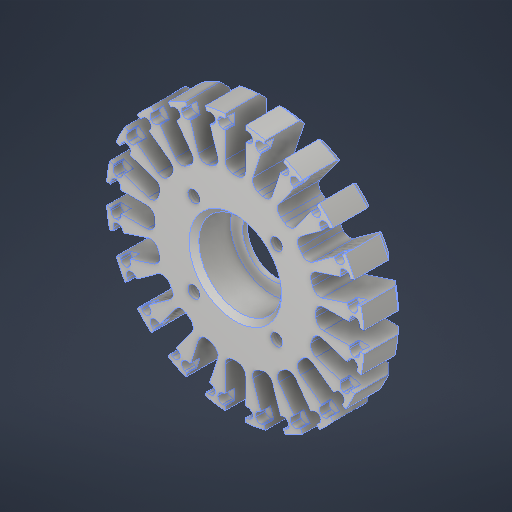
# Autodesk Inventor part: Radkasten
Saved by Autodesk Inventor 2025.2 (Build 292293000, 293)
## iProperties
Part Number: Radkasten
Material: Aluminium 6061
Document SubType Name: Modeling
Designer: rYan
Density: 2.7 g/cm^3
Appearance: Aluminium - flach
Mass: 11.5434 g
Surface Area: 96.0365 cm^2
Volume: 11.5434 cm^3
Author: rYan
Autodesk Inventor part; units mm, degrees
ref_plane "YZ Plane" through (0, 0, 0) normal (1, 0, 0) x (0, 1, 0)
ref_plane "XZ Plane" through (0, 0, 0) normal (0, 1, 0) x (-1, 0, 0)
ref_plane "XY Plane" through (0, 0, 0) normal (0, 0, 1) x (1, 0, 0)
sketch "Skizze1" plane through (0, 0, 0) normal (0, 0, 1) x (1, 0, 0)
  line L0 (0, 0) -> (0, 8.5)
  line L1 (4.75, 0) -> (4.75, 8.5)
  line L2 (4.75, 8.5) -> (5.8, 8.5)
  line L3 (5.8, 8.5) -> (5.8, 8.5)
  line L4 (21, 8.5) -> (26.5, 8.5)
  line L5 (26.5, 8.5) -> (26.5, 0)
  line L6 (26.5, 0) -> (4.75, 0)
  line L7 (-5.3, 0) -> (31.8, 0) projected
  line L8 (15.9, 8.5) -> (15.9, 8.5)
  line L9 (15.9, 8.5) -> (5.8, 8.5)
  line L10 (21, 8.5) -> (21, 8.5)
  line L11 (15.9, 8.5) -> (15.9, 8.5)
  line L12 (15.9, 8.5) -> (17.1, 8.5)
  line L13 (17.1, 8.5) -> (17.1, 8.5)
  line L14 (15.9, 8.5) -> (15.9, 8.5)
  line L15 (17.1, 8.5) -> (21, 8.5)
  line L16 (16.5, 8.5) -> (16.5, 0) construction
  dimension "d0" = 9.5
  dimension "d1" = 53
  dimension "d2" = 8.5
  dimension "d4" = 11.6
  dimension "d24" = 0
  dimension "d34" = 8.5
  dimension "d35" = 42
  dimension "d71" = 33
  dimension "d72" = 1.2
  dimension "d80" = 8.5
  constraints: 32 end point, 9 perpendicular, 4 point on line, 4 vertical, 3 horizontal, 2 midpoint, 1 collinear, 1 parallel
  measures "d0" diameter of L1 L0
  measures "d1" diameter of L5 L0
  measures "d2" distance of L4.end L5.end
  measures "d4" diameter of L3 L0
  measures "d24" distance of L8.start L8.end
  measures "d34" distance of L1.start L1.end
  measures "d35" diameter of L10 L0
  measures "d71" diameter of L16 L0
  measures "d72" distance of L11.end L12.end
  measures "d80" distance between parallel lines of L6 L12
revolve "Umdrehung1" add sketch "Skizze1" angle 360 about axis through (0, 0, 0) along (0, 1, 0)
sketch "Skizze2" plane through (0, 0, 0) normal (0, 1, 0) x (-1, 0, 0)
  circle A0 centre (0, 0) radius 26.5 projected
  circle A1 centre (0, 0) radius 16.5 construction
  line L0 (2.1, 26.5) -> (-2.1, 26.5)
  line L1 (-2.1, 26.5) -> (-2.1, 18.1)
  line L2 (-0.5, 16.5) -> (0.5, 16.5)
  line L3 (2.1, 18.1) -> (2.1, 26.5)
  line L4 (0, 0) -> (0, 26.5) construction
  arc A2 (0.5, 16.5) -> (2.1, 18.1) centre (0.5, 18.1) ccw
  arc A3 (-2.1, 18.1) -> (-0.5, 16.5) centre (-0.5, 18.1) ccw
  dimension "d6" = 1.6
  dimension "d7" = 4.2
  dimension "d8" = 33
  constraints: 10 end point, 5 tangent, 4 point on circle, 3 centre point, 2 parallel, 1 coincident, 1 equal radius, 1 horizontal, 1 midpoint, 1 perpendicular, 1 vertical, 1 vertical alignment, 2 other
  measures "d6" radius of A2
  measures "d7" distance between parallel lines of L1 L3
  measures "d8" diameter of A1
extrude "Querrolle" cut sketch "Skizze2" along normal blind 8.5 contours L3 A2 L2 A3 L1 A0 | A0 L0 L3 | L1 L0 A0 picked at (0, 20.9)
sketch "Skizze3" plane through (0, 0, 0) normal (0, 1, 0) x (-1, 0, 0)
  line L0 (2.6, 25.525) -> (-2.6, 25.525)
  line L1 (-3.6, 24.525) -> (-3.6, 24.475)
  line L2 (-2.6, 23.475) -> (2.6, 23.475)
  line L3 (3.6, 24.475) -> (3.6, 24.525)
  line L4 (0, -5.2833) -> (0, 31.7) projected
  line L5 (2.65, 25.504) -> (-2.65, 25.504) construction
  line L6 (-2.65, 25.504) -> (-2.65, 23.496) construction
  line L7 (-2.65, 23.496) -> (2.65, 23.496) construction
  line L8 (2.65, 23.496) -> (2.65, 25.504) construction
  line L9 (-2.65, 25.504) -> (-3, 25.4102) construction
  line L10 (-3, 25.4102) -> (-3, 23.5898) construction
  line L11 (-3, 23.5898) -> (-2.65, 23.496) construction
  line L12 (2.65, 25.504) -> (3, 25.4102) construction
  line L13 (3, 25.4102) -> (3, 23.5898) construction
  line L14 (3, 23.5898) -> (2.65, 23.496) construction
  line L15 (3, 24.5) -> (-3, 24.5) construction
  line L16 (0, 25.504) -> (0, 23.496) construction
  arc A0 (3.6, 24.525) -> (2.6, 25.525) centre (2.6, 24.525) ccw
  arc A1 (-2.6, 25.525) -> (-3.6, 24.525) centre (-2.6, 24.525) ccw
  arc A2 (-3.6, 24.475) -> (-2.6, 23.475) centre (-2.6, 24.475) ccw
  arc A3 (2.6, 23.475) -> (3.6, 24.475) centre (2.6, 24.475) ccw
  line L17 (3.6, 24.5) -> (-3.6, 24.5) construction
  line L18 (2.1, 18.1) -> (2.1, 26.4167) projected
  line L19 (3.375, 24.75) -> (2.6, 25.525) construction
  line L20 (2.6, 25.525) -> (-2.6, 25.525) construction
  line L21 (-2.6, 25.525) -> (-3.375, 24.75) construction
  line L22 (-3.375, 24.75) -> (-3.375, 24.5) construction
  line L23 (3.375, 24.75) -> (3.375, 24.5) construction
  line L24 (0, 24.5) -> (0, 31.35)
  circle A4 centre (0, 0) radius 31.35
  point P0 (3.6, 25.525)
  point P1 (-3.6, 25.525)
  point P2 (2.65, 24.5)
  point P3 (-2.65, 24.5)
  point P4 (0, 24.5)
  point P5 (2.1, 26.2538)
  dimension "d11" = 2.05
  dimension "d12" = 7.2
  dimension "d13" = 2.008
  dimension "d14" = 15
  dimension "d15" = 0.35
  dimension "d16" = 6
  dimension "d17" = 1
  dimension "d18" = 24.5
  dimension "d82" = 0.55
  dimension "d83" = 0.5
  dimension "d84" = 45
  dimension "d85" = 1.025
  dimension "d86" = 0.5
  dimension "d87" = 0.25
  dimension "d236" = 6.85
  constraints: 46 end point, 11 midpoint, 10 point on line, 8 point on circle, 8 tangent, 5 parallel, 4 centre point, 4 perpendicular, 3 equal radius, 3 horizontal, 1 coincident, 1 vertical, 1 vertical alignment, 8 other
  measures "d11" distance between parallel lines of L0 L2
  measures "d12" distance of point (3.6, 25.525) point (-3.6, 25.525)
  measures "d13" distance between parallel lines of L7 L5
  measures "d14" angle of L5 L9
  measures "d15" distance between parallel lines of L6 L10
  measures "d16" distance between parallel lines of L10 L13
  measures "d17" radius of A0
  measures "d18" distance from line of L17 point (0, 0)
  measures "d82" distance from line of L5.start L18
  measures "d83" distance from line of L0.start L18
  measures "d84" angle of L20 L21
  measures "d85" distance between parallel lines of L15 L20
  measures "d86" distance from line of L18 L19.end
  measures "d87" distance from line of L17 L19.start
  measures "d236" distance of L24.start L24.end
extrude "Achse" cut sketch "Skizze3" along normal blind 2 contours A0 L3 A3 L2 L18 L0 | L18 L2 L4 L0 | L4 L2 A2 L1 A1 L0
fillet "Rundung1" radius 0.1 4 edges at (-2.1, 1, 25.525) (-2.1, 1, 23.475) (2.1, 1, 25.525) (2.1, 1, 23.475)
pattern_circular "Runde Anordnung1" count 20 over 360 about axis through (0, -10, 0) along (0, 1, 0) of "Querrolle", "Achse", "Rundung1"
sketch "Skizze6" plane through (0.25, 8.5, 18) normal (0, -1, 0) x (0.7071068, 0, -0.7071068)
  circle A0 centre (12.5511, -12.9047) radius 8.5 construction
  line L0 (4.0511, -12.9047) -> (21.0511, -12.9047) construction
  line L1 (12.5511, -21.4047) -> (12.5511, -4.4047) construction
  dimension "d48" = 17
  constraints: 5 coincident, 4 end point, 4 midpoint, 4 point on circle, 1 centre point, 1 horizontal, 1 perpendicular
  measures "d48" diameter of A0
hole "Fräshilfe" [suppressed]
chamfer "Fasen" distance 1.5 angle 45 20 edges at (23.6117, 8.5, -12.0307) (18.7383, 8.5, -18.7383) (12.0307, 8.5, -23.6117) (4.1455, 8.5, -26.1737) (-4.1455, 8.5, -26.1737) (-12.0307, 8.5, -23.6117) (-18.7383, 8.5, -18.7383) (-23.6117, 8.5, -12.0307) (-26.1737, 8.5, -4.1455) (-26.1737, 8.5, 4.1455) (-23.6117, 8.5, 12.0307) (-18.7383, 8.5, 18.7383) (-12.0307, 8.5, 23.6117) (-4.1455, 8.5, 26.1737) (4.1455, 8.5, 26.1737) (12.0307, 8.5, 23.6117) (18.7383, 8.5, 18.7383) (23.6117, 8.5, 12.0307) (26.1737, 8.5, 4.1455) (26.1737, 8.5, -4.1455)
sketch "Skizze22" plane through (-24.9116, 8.5, -2.1) normal (0, 1, 0) x (1, 0, 0)
  line L0 (25.4822, 13.5146) -> (25.1616, 12.3978)
  arc A0 (25.1616, 12.3978) -> (24.6616, 12.3978) centre (24.9116, -2.1) ccw
  line L1 (24.6616, 12.3978) -> (24.3411, 13.5146)
  arc A1 (24.3411, 13.5146) -> (23.8469, 13.4887) centre (24.9116, -2.1) ccw
  line L2 (23.8469, 13.4887) -> (23.6448, 12.3446)
  arc A2 (23.6448, 12.3446) -> (23.1476, 12.2923) centre (24.9116, -2.1) ccw
  line L3 (23.1476, 12.2923) -> (22.7121, 13.3694)
  arc A3 (22.7121, 13.3694) -> (22.2233, 13.292) centre (24.9116, -2.1) ccw
  line L4 (22.2233, 13.292) -> (22.1419, 12.133)
  arc A4 (22.1419, 12.133) -> (21.6528, 12.0291) centre (24.9116, -2.1) ccw
  line L5 (21.6528, 12.0291) -> (21.1071, 13.0547)
  arc A5 (21.1071, 13.0547) -> (20.6291, 12.9267) centre (24.9116, -2.1) ccw
  line L6 (20.6291, 12.9267) -> (20.6693, 11.7655)
  arc A6 (20.6693, 11.7655) -> (20.1938, 11.611) centre (24.9116, -2.1) ccw
  line L7 (20.1938, 11.611) -> (19.5439, 12.574)
  arc A7 (19.5439, 12.574) -> (19.0818, 12.3967) centre (24.9116, -2.1) ccw
  line L8 (19.0818, 12.3967) -> (19.2432, 11.2461)
  arc A8 (19.2432, 11.2461) -> (18.7865, 11.0428) centre (24.9116, -2.1) ccw
  line L9 (18.7865, 11.0428) -> (18.0394, 11.9326)
  arc A9 (18.0394, 11.9326) -> (17.5984, 11.7079) centre (24.9116, -2.1) ccw
  line L10 (17.5984, 11.7079) -> (17.8792, 10.5805)
  arc A10 (17.8792, 10.5805) -> (17.4462, 10.3305) centre (24.9116, -2.1) ccw
  line L11 (17.4462, 10.3305) -> (16.6103, 11.1374)
  arc A11 (16.6103, 11.1374) -> (16.1952, 10.8678) centre (24.9116, -2.1) ccw
  line L12 (16.1952, 10.8678) -> (16.5923, 9.7759)
  arc A12 (16.5923, 9.7759) -> (16.1878, 9.4821) centre (24.9116, -2.1) ccw
  line L13 (16.1878, 9.4821) -> (15.2721, 10.1971)
  arc A13 (15.2721, 10.1971) -> (14.8874, 9.8857) centre (24.9116, -2.1) ccw
  line L14 (14.8874, 9.8857) -> (15.3965, 8.8413)
  arc A14 (15.3965, 8.8413) -> (15.0249, 8.5067) centre (24.9116, -2.1) ccw
  line L15 (15.0249, 8.5067) -> (14.0395, 9.1221)
  arc A15 (14.0395, 9.1221) -> (13.6895, 8.7722) centre (24.9116, -2.1) ccw
  line L16 (13.6895, 8.7722) -> (14.3049, 7.7867)
  arc A16 (14.3049, 7.7867) -> (13.9704, 7.4152) centre (24.9116, -2.1) ccw
  line L17 (13.9704, 7.4152) -> (12.926, 7.9242)
  arc A17 (12.926, 7.9242) -> (12.6145, 7.5396) centre (24.9116, -2.1) ccw
  line L18 (12.6145, 7.5396) -> (13.3296, 6.6239)
  arc A18 (13.3296, 6.6239) -> (13.0357, 6.2194) centre (24.9116, -2.1) ccw
  line L19 (13.0357, 6.2194) -> (11.9438, 6.6165)
  arc A19 (11.9438, 6.6165) -> (11.6743, 6.2014) centre (24.9116, -2.1) ccw
  line L20 (11.6743, 6.2014) -> (12.4811, 5.3654)
  arc A20 (12.4811, 5.3654) -> (12.2311, 4.9324) centre (24.9116, -2.1) ccw
  line L21 (12.2311, 4.9324) -> (11.1038, 5.2132)
  arc A21 (11.1038, 5.2132) -> (10.8791, 4.7722) centre (24.9116, -2.1) ccw
  line L22 (10.8791, 4.7722) -> (11.7689, 4.0252)
  arc A22 (11.7689, 4.0252) -> (11.5655, 3.5684) centre (24.9116, -2.1) ccw
  line L23 (11.5655, 3.5684) -> (10.415, 3.7298)
  arc A23 (10.415, 3.7298) -> (10.2376, 3.2678) centre (24.9116, -2.1) ccw
  line L24 (10.2376, 3.2678) -> (11.2006, 2.6178)
  arc A24 (11.2006, 2.6178) -> (11.0461, 2.1423) centre (24.9116, -2.1) ccw
  line L25 (11.0461, 2.1423) -> (9.885, 2.1826)
  arc A25 (9.885, 2.1826) -> (9.7569, 1.7045) centre (24.9116, -2.1) ccw
  line L26 (9.7569, 1.7045) -> (10.7826, 1.1588)
  arc A26 (10.7826, 1.1588) -> (10.6786, 0.6697) centre (24.9116, -2.1) ccw
  line L27 (10.6786, 0.6697) -> (9.5197, 0.5884)
  arc A27 (9.5197, 0.5884) -> (9.4422, 0.0996) centre (24.9116, -2.1) ccw
  line L28 (9.4422, 0.0996) -> (10.5194, -0.3359)
  arc A28 (10.5194, -0.3359) -> (10.4671, -0.8332) centre (24.9116, -2.1) ccw
  line L29 (10.4671, -0.8332) -> (9.323, -1.0352)
  arc A29 (9.323, -1.0352) -> (9.2971, -1.5295) centre (24.9116, -2.1) ccw
  line L30 (9.2971, -1.5295) -> (10.4138, -1.85)
  arc A30 (10.4138, -1.85) -> (10.4138, -2.35) centre (24.9116, -2.1) ccw
  line L31 (10.4138, -2.35) -> (9.2971, -2.6705)
  arc A31 (9.2971, -2.6705) -> (9.323, -3.1648) centre (24.9116, -2.1) ccw
  line L32 (9.323, -3.1648) -> (10.4671, -3.3668)
  arc A32 (10.4671, -3.3668) -> (10.5194, -3.8641) centre (24.9116, -2.1) ccw
  line L33 (10.5194, -3.8641) -> (9.4422, -4.2996)
  arc A33 (9.4422, -4.2996) -> (9.5197, -4.7884) centre (24.9116, -2.1) ccw
  line L34 (9.5197, -4.7884) -> (10.6786, -4.8697)
  arc A34 (10.6786, -4.8697) -> (10.7826, -5.3588) centre (24.9116, -2.1) ccw
  line L35 (10.7826, -5.3588) -> (9.7569, -5.9045)
  arc A35 (9.7569, -5.9045) -> (9.885, -6.3826) centre (24.9116, -2.1) ccw
  line L36 (9.885, -6.3826) -> (11.0461, -6.3423)
  arc A36 (11.0461, -6.3423) -> (11.2006, -6.8178) centre (24.9116, -2.1) ccw
  line L37 (11.2006, -6.8178) -> (10.2376, -7.4678)
  arc A37 (10.2376, -7.4678) -> (10.415, -7.9298) centre (24.9116, -2.1) ccw
  line L38 (10.415, -7.9298) -> (11.5655, -7.7684)
  arc A38 (11.5655, -7.7684) -> (11.7689, -8.2252) centre (24.9116, -2.1) ccw
  line L39 (11.7689, -8.2252) -> (10.8791, -8.9722)
  arc A39 (10.8791, -8.9722) -> (11.1038, -9.4132) centre (24.9116, -2.1) ccw
  line L40 (11.1038, -9.4132) -> (12.2311, -9.1324)
  arc A40 (12.2311, -9.1324) -> (12.4811, -9.5654) centre (24.9116, -2.1) ccw
  line L41 (12.4811, -9.5654) -> (11.6743, -10.4014)
  arc A41 (11.6743, -10.4014) -> (11.9438, -10.8165) centre (24.9116, -2.1) ccw
  line L42 (11.9438, -10.8165) -> (13.0357, -10.4194)
  arc A42 (13.0357, -10.4194) -> (13.3296, -10.8239) centre (24.9116, -2.1) ccw
  line L43 (13.3296, -10.8239) -> (12.6145, -11.7396)
  arc A43 (12.6145, -11.7396) -> (12.926, -12.1242) centre (24.9116, -2.1) ccw
  line L44 (12.926, -12.1242) -> (13.9704, -11.6152)
  arc A44 (13.9704, -11.6152) -> (14.3049, -11.9867) centre (24.9116, -2.1) ccw
  line L45 (14.3049, -11.9867) -> (13.6895, -12.9722)
  arc A45 (13.6895, -12.9722) -> (14.0395, -13.3221) centre (24.9116, -2.1) ccw
  line L46 (14.0395, -13.3221) -> (15.0249, -12.7067)
  arc A46 (15.0249, -12.7067) -> (15.3965, -13.0413) centre (24.9116, -2.1) ccw
  line L47 (15.3965, -13.0413) -> (14.8874, -14.0857)
  arc A47 (14.8874, -14.0857) -> (15.2721, -14.3971) centre (24.9116, -2.1) ccw
  line L48 (15.2721, -14.3971) -> (16.1878, -13.6821)
  arc A48 (16.1878, -13.6821) -> (16.5923, -13.9759) centre (24.9116, -2.1) ccw
  line L49 (16.5923, -13.9759) -> (16.1952, -15.0678)
  arc A49 (16.1952, -15.0678) -> (16.6103, -15.3374) centre (24.9116, -2.1) ccw
  line L50 (16.6103, -15.3374) -> (17.4462, -14.5305)
  arc A50 (17.4462, -14.5305) -> (17.8792, -14.7805) centre (24.9116, -2.1) ccw
  line L51 (17.8792, -14.7805) -> (17.5984, -15.9079)
  arc A51 (17.5984, -15.9079) -> (18.0394, -16.1326) centre (24.9116, -2.1) ccw
  line L52 (18.0394, -16.1326) -> (18.7865, -15.2428)
  arc A52 (18.7865, -15.2428) -> (19.2432, -15.4461) centre (24.9116, -2.1) ccw
  line L53 (19.2432, -15.4461) -> (19.0818, -16.5967)
  arc A53 (19.0818, -16.5967) -> (19.5439, -16.774) centre (24.9116, -2.1) ccw
  line L54 (19.5439, -16.774) -> (20.1938, -15.811)
  arc A54 (20.1938, -15.811) -> (20.6693, -15.9655) centre (24.9116, -2.1) ccw
  line L55 (20.6693, -15.9655) -> (20.6291, -17.1267)
  arc A55 (20.6291, -17.1267) -> (21.1071, -17.2547) centre (24.9116, -2.1) ccw
  line L56 (21.1071, -17.2547) -> (21.6528, -16.2291)
  arc A56 (21.6528, -16.2291) -> (22.1419, -16.333) centre (24.9116, -2.1) ccw
  line L57 (22.1419, -16.333) -> (22.2233, -17.492)
  arc A57 (22.2233, -17.492) -> (22.7121, -17.5694) centre (24.9116, -2.1) ccw
  line L58 (22.7121, -17.5694) -> (23.1476, -16.4923)
  arc A58 (23.1476, -16.4923) -> (23.6448, -16.5446) centre (24.9116, -2.1) ccw
  line L59 (23.6448, -16.5446) -> (23.8469, -17.6887)
  arc A59 (23.8469, -17.6887) -> (24.3411, -17.7146) centre (24.9116, -2.1) ccw
  line L60 (24.3411, -17.7146) -> (24.6616, -16.5978)
  arc A60 (24.6616, -16.5978) -> (25.1616, -16.5978) centre (24.9116, -2.1) ccw
  line L61 (25.1616, -16.5978) -> (25.4822, -17.7146)
  arc A61 (25.4822, -17.7146) -> (25.9764, -17.6887) centre (24.9116, -2.1) ccw
  line L62 (25.9764, -17.6887) -> (26.1785, -16.5446)
  arc A62 (26.1785, -16.5446) -> (26.6757, -16.4923) centre (24.9116, -2.1) ccw
  line L63 (26.6757, -16.4923) -> (27.1112, -17.5694)
  arc A63 (27.1112, -17.5694) -> (27.6, -17.492) centre (24.9116, -2.1) ccw
  line L64 (27.6, -17.492) -> (27.6814, -16.333)
  arc A64 (27.6814, -16.333) -> (28.1705, -16.2291) centre (24.9116, -2.1) ccw
  line L65 (28.1705, -16.2291) -> (28.7162, -17.2547)
  arc A65 (28.7162, -17.2547) -> (29.1942, -17.1267) centre (24.9116, -2.1) ccw
  line L66 (29.1942, -17.1267) -> (29.154, -15.9655)
  arc A66 (29.154, -15.9655) -> (29.6295, -15.811) centre (24.9116, -2.1) ccw
  line L67 (29.6295, -15.811) -> (30.2794, -16.774)
  arc A67 (30.2794, -16.774) -> (30.7415, -16.5967) centre (24.9116, -2.1) ccw
  line L68 (30.7415, -16.5967) -> (30.5801, -15.4461)
  arc A68 (30.5801, -15.4461) -> (31.0368, -15.2428) centre (24.9116, -2.1) ccw
  line L69 (31.0368, -15.2428) -> (31.7839, -16.1326)
  arc A69 (31.7839, -16.1326) -> (32.2248, -15.9079) centre (24.9116, -2.1) ccw
  line L70 (32.2248, -15.9079) -> (31.9441, -14.7805)
  arc A70 (31.9441, -14.7805) -> (32.3771, -14.5305) centre (24.9116, -2.1) ccw
  line L71 (32.3771, -14.5305) -> (33.213, -15.3374)
  arc A71 (33.213, -15.3374) -> (33.6281, -15.0678) centre (24.9116, -2.1) ccw
  line L72 (33.6281, -15.0678) -> (33.231, -13.9759)
  arc A72 (33.231, -13.9759) -> (33.6355, -13.6821) centre (24.9116, -2.1) ccw
  line L73 (33.6355, -13.6821) -> (34.5512, -14.3971)
  arc A73 (34.5512, -14.3971) -> (34.9359, -14.0857) centre (24.9116, -2.1) ccw
  line L74 (34.9359, -14.0857) -> (34.4268, -13.0413)
  arc A74 (34.4268, -13.0413) -> (34.7984, -12.7067) centre (24.9116, -2.1) ccw
  line L75 (34.7984, -12.7067) -> (35.7838, -13.3221)
  arc A75 (35.7838, -13.3221) -> (36.1338, -12.9722) centre (24.9116, -2.1) ccw
  line L76 (36.1338, -12.9722) -> (35.5184, -11.9867)
  arc A76 (35.5184, -11.9867) -> (35.8529, -11.6152) centre (24.9116, -2.1) ccw
  line L77 (35.8529, -11.6152) -> (36.8973, -12.1242)
  arc A77 (36.8973, -12.1242) -> (37.2088, -11.7396) centre (24.9116, -2.1) ccw
  line L78 (37.2088, -11.7396) -> (36.4937, -10.8239)
  arc A78 (36.4937, -10.8239) -> (36.7876, -10.4194) centre (24.9116, -2.1) ccw
  line L79 (36.7876, -10.4194) -> (37.8795, -10.8165)
  arc A79 (37.8795, -10.8165) -> (38.149, -10.4014) centre (24.9116, -2.1) ccw
  line L80 (38.149, -10.4014) -> (37.3421, -9.5654)
  arc A80 (37.3421, -9.5654) -> (37.5921, -9.1324) centre (24.9116, -2.1) ccw
  line L81 (37.5921, -9.1324) -> (38.7195, -9.4132)
  arc A81 (38.7195, -9.4132) -> (38.9442, -8.9722) centre (24.9116, -2.1) ccw
  line L82 (38.9442, -8.9722) -> (38.0544, -8.2252)
  arc A82 (38.0544, -8.2252) -> (38.2578, -7.7684) centre (24.9116, -2.1) ccw
  line L83 (38.2578, -7.7684) -> (39.4083, -7.9298)
  arc A83 (39.4083, -7.9298) -> (39.5857, -7.4678) centre (24.9116, -2.1) ccw
  line L84 (39.5857, -7.4678) -> (38.6227, -6.8178)
  arc A84 (38.6227, -6.8178) -> (38.7772, -6.3423) centre (24.9116, -2.1) ccw
  line L85 (38.7772, -6.3423) -> (39.9383, -6.3826)
  arc A85 (39.9383, -6.3826) -> (40.0664, -5.9045) centre (24.9116, -2.1) ccw
  line L86 (40.0664, -5.9045) -> (39.0407, -5.3588)
  arc A86 (39.0407, -5.3588) -> (39.1447, -4.8697) centre (24.9116, -2.1) ccw
  line L87 (39.1447, -4.8697) -> (40.3036, -4.7884)
  arc A87 (40.3036, -4.7884) -> (40.381, -4.2996) centre (24.9116, -2.1) ccw
  line L88 (40.381, -4.2996) -> (39.3039, -3.8641)
  arc A88 (39.3039, -3.8641) -> (39.3562, -3.3668) centre (24.9116, -2.1) ccw
  line L89 (39.3562, -3.3668) -> (40.5003, -3.1648)
  arc A89 (40.5003, -3.1648) -> (40.5262, -2.6705) centre (24.9116, -2.1) ccw
  line L90 (40.5262, -2.6705) -> (39.4095, -2.35)
  arc A90 (39.4095, -2.35) -> (39.4095, -1.85) centre (24.9116, -2.1) ccw
  line L91 (39.4095, -1.85) -> (40.5262, -1.5295)
  arc A91 (40.5262, -1.5295) -> (40.5003, -1.0352) centre (24.9116, -2.1) ccw
  line L92 (40.5003, -1.0352) -> (39.3562, -0.8332)
  arc A92 (39.3562, -0.8332) -> (39.3039, -0.3359) centre (24.9116, -2.1) ccw
  line L93 (39.3039, -0.3359) -> (40.381, 0.0996)
  arc A93 (40.381, 0.0996) -> (40.3036, 0.5884) centre (24.9116, -2.1) ccw
  line L94 (40.3036, 0.5884) -> (39.1447, 0.6697)
  arc A94 (39.1447, 0.6697) -> (39.0407, 1.1588) centre (24.9116, -2.1) ccw
  line L95 (39.0407, 1.1588) -> (40.0664, 1.7045)
  arc A95 (40.0664, 1.7045) -> (39.9383, 2.1826) centre (24.9116, -2.1) ccw
  line L96 (39.9383, 2.1826) -> (38.7772, 2.1423)
  arc A96 (38.7772, 2.1423) -> (38.6227, 2.6178) centre (24.9116, -2.1) ccw
  line L97 (38.6227, 2.6178) -> (39.5857, 3.2678)
  arc A97 (39.5857, 3.2678) -> (39.4083, 3.7298) centre (24.9116, -2.1) ccw
  line L98 (39.4083, 3.7298) -> (38.2578, 3.5684)
  arc A98 (38.2578, 3.5684) -> (38.0544, 4.0252) centre (24.9116, -2.1) ccw
  line L99 (38.0544, 4.0252) -> (38.9442, 4.7722)
  arc A99 (38.9442, 4.7722) -> (38.7195, 5.2132) centre (24.9116, -2.1) ccw
  line L100 (38.7195, 5.2132) -> (37.5921, 4.9324)
  arc A100 (37.5921, 4.9324) -> (37.3421, 5.3654) centre (24.9116, -2.1) ccw
  line L101 (37.3421, 5.3654) -> (38.149, 6.2014)
  arc A101 (38.149, 6.2014) -> (37.8795, 6.6165) centre (24.9116, -2.1) ccw
  line L102 (37.8795, 6.6165) -> (36.7876, 6.2194)
  arc A102 (36.7876, 6.2194) -> (36.4937, 6.6239) centre (24.9116, -2.1) ccw
  line L103 (36.4937, 6.6239) -> (37.2088, 7.5396)
  arc A103 (37.2088, 7.5396) -> (36.8973, 7.9242) centre (24.9116, -2.1) ccw
  line L104 (36.8973, 7.9242) -> (35.8529, 7.4152)
  arc A104 (35.8529, 7.4152) -> (35.5184, 7.7867) centre (24.9116, -2.1) ccw
  line L105 (35.5184, 7.7867) -> (36.1338, 8.7722)
  arc A105 (36.1338, 8.7722) -> (35.7838, 9.1221) centre (24.9116, -2.1) ccw
  line L106 (35.7838, 9.1221) -> (34.7984, 8.5067)
  arc A106 (34.7984, 8.5067) -> (34.4268, 8.8413) centre (24.9116, -2.1) ccw
  line L107 (34.4268, 8.8413) -> (34.9359, 9.8857)
  arc A107 (34.9359, 9.8857) -> (34.5512, 10.1971) centre (24.9116, -2.1) ccw
  line L108 (34.5512, 10.1971) -> (33.6355, 9.4821)
  arc A108 (33.6355, 9.4821) -> (33.231, 9.7759) centre (24.9116, -2.1) ccw
  line L109 (33.231, 9.7759) -> (33.6281, 10.8678)
  arc A109 (33.6281, 10.8678) -> (33.213, 11.1374) centre (24.9116, -2.1) ccw
  line L110 (33.213, 11.1374) -> (32.3771, 10.3305)
  arc A110 (32.3771, 10.3305) -> (31.9441, 10.5805) centre (24.9116, -2.1) ccw
  line L111 (31.9441, 10.5805) -> (32.2248, 11.7079)
  arc A111 (32.2248, 11.7079) -> (31.7839, 11.9326) centre (24.9116, -2.1) ccw
  line L112 (31.7839, 11.9326) -> (31.0368, 11.0428)
  arc A112 (31.0368, 11.0428) -> (30.5801, 11.2461) centre (24.9116, -2.1) ccw
  line L113 (30.5801, 11.2461) -> (30.7415, 12.3967)
  arc A113 (30.7415, 12.3967) -> (30.2794, 12.574) centre (24.9116, -2.1) ccw
  line L114 (30.2794, 12.574) -> (29.6295, 11.611)
  arc A114 (29.6295, 11.611) -> (29.154, 11.7655) centre (24.9116, -2.1) ccw
  line L115 (29.154, 11.7655) -> (29.1942, 12.9267)
  arc A115 (29.1942, 12.9267) -> (28.7162, 13.0547) centre (24.9116, -2.1) ccw
  line L116 (28.7162, 13.0547) -> (28.1705, 12.0291)
  arc A116 (28.1705, 12.0291) -> (27.6814, 12.133) centre (24.9116, -2.1) ccw
  line L117 (27.6814, 12.133) -> (27.6, 13.292)
  arc A117 (27.6, 13.292) -> (27.1112, 13.3694) centre (24.9116, -2.1) ccw
  line L118 (27.1112, 13.3694) -> (26.6757, 12.2923)
  arc A118 (26.6757, 12.2923) -> (26.1785, 12.3446) centre (24.9116, -2.1) ccw
  line L119 (26.1785, 12.3446) -> (25.9764, 13.4887)
  arc A119 (25.9764, 13.4887) -> (25.4822, 13.5146) centre (24.9116, -2.1) ccw
  point P0 (24.9116, -2.1)
  point P1 (24.9116, -2.1)
  point P2 (48.0004, 1.5569)
  point P3 (21.2547, 20.9887)
  point P4 (1.8229, -5.7569)
  point P5 (28.5685, -25.1887)
  dimension "d207" = 360
  constraints: 240 end point, 240 point on circle, 120 centre point, 5 other
hole "Bohrung4" at (23.0887, 8.5, -3.6569) at (-3.6569, 8.5, -23.0887) at (-23.0887, 8.5, 3.6569) at (3.6569, 8.5, 23.0887) direction (0, -1, 0) diameter 1.567 depth 4 tip angle 118 thread size "M2x0.4" class "6H" standard "ISO Metric profile"
sketch "Skizze23" plane through (0.5, 0, 18.1) normal (0, -1, 0) x (0.7071068, 0, -0.7071068)
  circle A0 centre (12.4451, -13.1522) radius 7.05
  dimension "d216" = 14.1
  constraints: 1 centre point, 1 coincident
  measures "d216" diameter of A0
extrude "Extrusion16" cut sketch "Skizze23" against normal blind 7.5
sketch "Skizze24" plane through (0.5, 0, 18.1) normal (0, -1, 0) x (0.7071068, 0, -0.7071068)
  circle A0 centre (12.4451, -13.1522) radius 8.5
  dimension "d219" = 17
  constraints: 1 centre point, 1 coincident
  measures "d219" diameter of A0
extrude "Extrusion17" cut sketch "Skizze24" against normal blind 7.5
chamfer "Fasen26" distance 1 angle 45 1 edges at (-6.0104, 0, 6.0104)
sketch "Skizze25" plane through (0.5, 0, 18.1) normal (0, -1, 0) x (0.7071068, 0, -0.7071068)
  circle A0 centre (12.4451, -13.1522) radius 12 construction
  line L0 (12.4451, -1.1522) -> (12.4451, -25.1522) construction
  line L1 (0.4451, -13.1522) -> (24.4451, -13.1522) construction
  point P0 (12.4451, -13.1522)
  dimension "d225" = 24
  constraints: 5 coincident, 4 end point, 4 point on circle, 3 midpoint, 1 centre point, 1 perpendicular, 1 vertical
  measures "d225" diameter of A0
hole "Bohrung5" at (-8.4853, 0, -8.4853) at (-8.4853, 0, 8.4853) at (8.4853, 0, 8.4853) at (8.4853, 0, -8.4853) direction (0, 1, 0) diameter 2.459 depth 6 tip angle 118 thread size "M3x0.5" class "6H" standard "ISO Metric profile"
sketch "Skizze26" plane through (0, 7.5, 0) normal (0, -1, 0) x (1, 0, 0)
  circle A0 centre (0, 0) radius 6
  dimension "d233" = 12
  constraints: 1 centre point, 1 coincident
  measures "d233" diameter of A0
extrude "Extrusion18" cut sketch "Skizze26" against normal blind 10
